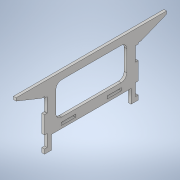
# Autodesk Inventor part: open_case
Saved by Autodesk Inventor 2020 (Build 240168000, 168)
## iProperties
Created: 2019-12-18
Part Number: open_case
Material: Generic
Document SubType Name: Modeling
Designer: fabfarm
Density: 1 g/cm^3
Appearance: Default
Author: fabfarm
Autodesk Inventor part; units mm, degrees
ref_plane "YZ Plane" through (0, 0, 0) normal (1, 0, 0) x (0, 1, 0)
ref_plane "XZ Plane" through (0, 0, 0) normal (0, 1, 0) x (-1, 0, 0)
ref_plane "XY Plane" through (0, 0, 0) normal (0, 0, 1) x (1, 0, 0)
sketch "Sketch1" plane through (0, 0, 0) normal (1, 0, 0) x (0, 1, 0)
  line L0 (-163.875, -330) -> (163.875, -330)
  line L1 (163.875, -330) -> (163.875, 330)
  line L2 (163.875, 330) -> (-163.875, 330)
  line L3 (-163.875, 330) -> (-163.875, -330)
  line L4 (-163.875, -330) -> (163.875, 330) construction
  line L5 (163.875, -330) -> (-163.875, 330) construction
  point P0 (0, 0)
  dimension "d0" = 660
  dimension "d1" = 327.75
  constraints: 12 end point, 2 midpoint, 2 parallel, 1 horizontal, 1 perpendicular
  measures "d0" distance of L0.end L1.end
  measures "d1" distance of L0.start L0.end
extrude "Extrusion1" add sketch "Sketch1" along normal blind 18.55
sketch "Sketch2" plane through (18.55, 0, 0) normal (1, 0, 0) x (0, 0, -1)
  line L0 (-330, 163.875) -> (-330, -163.875) projected
  line L1 (-330, 61.225) -> (-311.45, 61.225)
  line L2 (-311.45, 61.225) -> (-311.45, -38.975)
  line L3 (-311.45, -38.975) -> (-330, -38.975)
  line L4 (-330, -38.975) -> (-330, 61.225)
  line L5 (330, 163.875) -> (-330, 163.875) projected
  line L6 (-330, -163.875) -> (330, -163.875) projected
  dimension "d20" = 100.2
  dimension "d21" = 102.65
  dimension "d22" = 124.9
  dimension "d23" = 18.55
  constraints: 8 end point, 2 parallel, 1 horizontal, 1 perpendicular, 1 point on line
  measures "d20" distance of L1.end L2.end
  measures "d21" distance from line of L5 L1.end
  measures "d22" distance between parallel lines of L6 L3
  measures "d23" distance of L1.start L1.end
extrude "Extrusion2" cut sketch "Sketch2" against normal blind 18.55
mirror "Mirror1" about plane through (0, 0, 0) normal (0, 0, 1) of "Extrusion2"
sketch "Sketch3" plane through (18.55, 0, 0) normal (1, 0, 0) x (0, 0, -1)
  line L0 (210, -113.875) -> (-210, -113.875)
  line L1 (-250, -73.875) -> (-250, 73.875)
  line L2 (-210, 113.875) -> (210, 113.875)
  line L3 (250, 73.875) -> (250, -73.875)
  line L4 (250, -113.875) -> (-250, 113.875) construction
  line L5 (-250, -113.875) -> (250, 113.875) construction
  arc A0 (-210, 113.875) -> (-250, 73.875) centre (-210, 73.875) ccw
  arc A1 (-250, -73.875) -> (-210, -113.875) centre (-210, -73.875) ccw
  arc A2 (250, 73.875) -> (210, 113.875) centre (210, 73.875) ccw
  arc A3 (210, -113.875) -> (250, -73.875) centre (210, -73.875) ccw
  line L6 (-330, -38.975) -> (-330, -163.875) projected
  line L7 (330, 163.875) -> (-330, 163.875) projected
  point P0 (0, 0)
  dimension "d17" = 40
  dimension "d40" = 80
  dimension "d41" = 50
  constraints: 12 end point, 8 point on circle, 8 point on line, 8 tangent, 4 centre point, 3 equal radius, 2 midpoint, 2 parallel, 1 horizontal, 1 perpendicular
  measures "d17" radius of A0
  measures "d40" distance between parallel lines of L6 L1
  measures "d41" distance between parallel lines of L7 L2
extrude "Extrusion3" cut sketch "Sketch3" against normal blind 18.55
sketch "Esquisse4" plane through (18.55, 0, 0) normal (1, 0, 0) x (0, 0, -1)
  circle A0 centre (-312.5725, 60.1025) radius 1.5875
  circle A1 centre (-312.5725, -37.8525) radius 1.5875
  line L0 (-312.5725, 60.1025) -> (-311.45, 61.225) construction
  line L1 (-311.45, 61.225) -> (-311.45, -38.975) projected
  line L2 (210, 113.875) -> (-210, 113.875) projected
  line L3 (0, 113.875) -> (0, -113.875) construction
  line L4 (-210, -113.875) -> (210, -113.875) projected
  circle A2 centre (312.5725, 60.1025) radius 1.5875
  circle A3 centre (312.5725, -37.8525) radius 1.5875
  line L5 (312.5725, 60.1025) -> (311.45, 61.225) construction
  point P0 (0, 0)
  point P1 (311.45, 61.225)
  point P2 (311.45, -38.975)
  point P3 (311.45, -38.975)
  dimension "d24" = 3.175
  dimension "d39" = 45
  constraints: 6 end point, 4 symmetric about line, 2 midpoint, 2 vertical, 1 vertical alignment, 12 other
  measures "d39" angle of L1 L0
extrude "Extrusion4" cut sketch "Esquisse4" against normal blind 18.55
sketch "Esquisse5" plane through (18.55, 0, 0) normal (1, 0, 0) x (0, 0, -1)
  line L0 (-211.5, -163.875) -> (-111.4, -163.875)
  line L1 (-111.4, -163.875) -> (-111.4, -145.225)
  line L2 (-111.4, -145.225) -> (-211.5, -145.225)
  line L3 (-211.5, -145.225) -> (-211.5, -163.875)
  line L4 (111.4, -163.875) -> (211.5, -163.875)
  line L5 (211.5, -163.875) -> (211.5, -145.225)
  line L6 (211.5, -145.225) -> (111.4, -145.225)
  line L7 (111.4, -145.225) -> (111.4, -163.875)
  line L8 (-330, -38.975) -> (-330, -163.875) projected
  line L9 (330, -163.875) -> (330, -38.975) projected
  line L10 (210, -113.875) -> (-210, -113.875) projected
  line L11 (-330, -163.875) -> (330, -163.875) projected
  point P0 (0, 0)
  dimension "d27" = 100.1
  dimension "d28" = 100.1
  dimension "d29" = 118.5
  dimension "d30" = 118.5
  dimension "d38" = 18.65
  constraints: 16 end point, 4 parallel, 2 collinear, 2 horizontal, 2 perpendicular, 1 point on line
  measures "d27" distance of L1.end L2.end
  measures "d28" distance of L5.end L6.end
  measures "d29" distance between parallel lines of L8 L3
  measures "d30" distance between parallel lines of L9 L5
  measures "d38" distance of L0.end L1.end
extrude "Extrusion5" cut sketch "Esquisse5" against normal blind 20
sketch "Esquisse6" plane through (18.55, 0, 0) normal (1, 0, 0) x (0, 0, -1)
  circle A0 centre (-210.3686, -146.3564) radius 1.6
  circle A1 centre (-112.5314, -146.3564) radius 1.6
  line L0 (-211.5, -163.875) -> (-211.5, -145.225) projected
  line L1 (-211.5, -145.225) -> (-210.3686, -146.3564) construction
  circle A2 centre (112.5314, -146.3564) radius 1.6
  circle A3 centre (210.3686, -146.3564) radius 1.6
  point P0 (0, 0)
  point P1 (-111.4, -145.225)
  point P2 (111.4, -145.225)
  point P3 (211.5, -145.225)
  dimension "d42" = 3.2
  dimension "d43" = 45
  constraints: 3 horizontal alignment, 2 end point, 12 other
  measures "d43" angle of L0 L1
extrude "Extrusion6" cut sketch "Esquisse6" against normal blind 20
sketch "Esquisse8" plane through (18.55, 0, 0) normal (1, 0, 0) x (0, 0, -1)
  line L0 (-330, -38.975) -> (-330, -163.875) projected
  line L1 (-330, -163.875) -> (330, -163.875)
  line L2 (330, -163.875) -> (330, -181.7314)
  line L3 (280, -183.875) -> (-280, -183.875)
  line L4 (-330, -183.875) -> (-330, -163.875)
  line L5 (330, -163.875) -> (330, -38.975) projected
  line L6 (-280, -183.875) -> (-280, -280.325)
  line L7 (-280, -280.325) -> (-330, -280.325)
  line L8 (-330, -280.325) -> (-330, -183.875)
  line L9 (280, -183.875) -> (280, -280.325)
  line L10 (280, -280.325) -> (330, -280.325)
  line L11 (330, -280.325) -> (330, -181.7314)
  point P0 (0, 0)
  dimension "d45" = 20
  dimension "d46" = 116.45
  dimension "d47" = 50
  constraints: 20 end point, 4 parallel, 3 collinear, 2 vertical, 1 horizontal, 1 perpendicular, 1 point on line
  measures "d45" distance between parallel lines of L1 L3
  measures "d46" distance between parallel lines of L7 L1
  measures "d47" distance of L6.end L7.end
extrude "Extrusion7" add sketch "Esquisse8" against normal blind 18.55
sketch "Esquisse9" plane through (18.55, 0, 0) normal (1, 0, 0) x (0, 0, -1)
  line L0 (-330, -248.875) -> (-311.35, -248.875)
  line L1 (-311.35, -248.875) -> (-311.35, -163.675)
  line L2 (-311.35, -163.675) -> (-330, -163.675)
  line L3 (-330, -163.675) -> (-330, -248.875)
  line L4 (330, -248.875) -> (311.35, -248.875)
  line L5 (311.35, -248.875) -> (311.35, -163.675)
  line L6 (311.35, -163.675) -> (330, -163.675)
  line L7 (330, -163.675) -> (330, -248.875)
  line L8 (330, -280.325) -> (330, -38.975) projected
  line L9 (-330, -38.975) -> (-330, -280.325) projected
  line L10 (-330, -280.325) -> (-280, -280.325) projected
  point P0 (0, 0)
  dimension "d50" = 85.2
  dimension "d51" = 31.45
  dimension "d52" = 18.65
  constraints: 16 end point, 5 collinear, 4 parallel, 2 horizontal, 2 perpendicular
  measures "d50" distance of L4.end L5.end
  measures "d51" distance between parallel lines of L10 L0
  measures "d52" distance of L0.start L0.end
extrude "Extrusion8" cut sketch "Esquisse9" against normal blind 18.55
sketch "Esquisse10" plane through (18.55, 0, 0) normal (1, 0, 0) x (0, 0, -1)
  line L0 (-330, 163.875) -> (-330, 61.225) projected
  line L1 (-330, 71.225) -> (-350, 71.225)
  line L2 (-530, 163.875) -> (-330, 163.875)
  line L3 (-530, 163.875) -> (-530, 143.875)
  line L4 (-530, 143.875) -> (-350, 71.225)
  line L5 (-330, 61.225) -> (-313.6951, 61.225) projected
  line L6 (330, 163.875) -> (-330, 163.875) projected
  line L7 (0, 163.875) -> (0, -183.875) construction
  line L8 (-280, -183.875) -> (280, -183.875) projected
  line L9 (-330, 163.875) -> (-330, 71.225)
  line L10 (330, 163.875) -> (330, 61.225)
  line L11 (330, 71.225) -> (350, 71.225)
  line L12 (530, 163.875) -> (330, 163.875)
  line L13 (530, 163.875) -> (530, 143.875)
  line L14 (530, 143.875) -> (350, 71.225)
  line L15 (330, 61.225) -> (313.6951, 61.225)
  line L16 (330, 163.875) -> (330, 71.225)
  point P0 (0, 0)
  dimension "d55" = 20
  dimension "d56" = 20
  dimension "d58" = 10
  dimension "d59" = 200
  constraints: 26 end point, 6 symmetric about line, 2 midpoint, 2 point on line, 1 collinear, 1 horizontal, 1 parallel, 1 vertical
  measures "d55" distance of L1.start L1.end
  measures "d56" distance of L2.start L3.end
  measures "d58" distance between parallel lines of L5 L1
  measures "d59" distance of L2.start L0.start
extrude "Extrusion9" add sketch "Esquisse10" against normal blind 18.55
body "Solid1"
